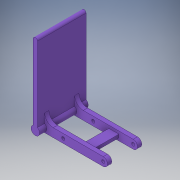
# Autodesk Inventor part: Mouth-Height-Lever-front
Saved by Autodesk Inventor 2018.3 (Build 223284000, 284)
## iProperties
Created: 2018-05-17
Part Number: Mouth-Height-Lever-front
Material: Generisch
Document SubType Name: Modeling
Designer: JochenAlt
Density: 1 g/cm^3
Appearance: Violett
Author: JochenAlt
Autodesk Inventor part; units mm, degrees
ref_plane "YZ Plane" through (0, 0, 0) normal (1, 0, 0) x (0, 1, 0)
ref_plane "XZ Plane" through (0, 0, 0) normal (0, 1, 0) x (-1, 0, 0)
ref_plane "XY Plane" through (0, 0, 0) normal (0, 0, 1) x (1, 0, 0)
sketch "Skizze4" plane through (0, 0, 0) normal (0, 1, 0) x (-1, 0, 0)
  line L0 (-45.5216, 3) -> (-3, 3) construction
  line L1 (0, -14.9) -> (0, 68.4) construction
  line L2 (-58.2259, 0) -> (9.7043, 0) construction
  circle A0 centre (-45.5216, 0) radius 3
  circle A1 centre (-45.5216, 0) radius 1.1
  circle A2 centre (-3, 0) radius 3
  line L3 (-12.1436, -3) -> (-45.5216, -3) construction
  line L4 (-45.5216, -3) -> (-17.5581, -3)
  line L5 (-1.5, 2.5981) -> (-1.5, 55)
  arc A3 (-1.5, 55) -> (-4.5, 55) centre (-3, 55) ccw
  circle A4 centre (-17.5581, 0) radius 1.1
  line L6 (-4.5, 9) -> (-4.5, 55)
  line L7 (-10.5, 3) -> (-3, 3)
  line L8 (-3, 0) -> (-3, 55) construction
  line L9 (-4.5, 9) -> (-4.5, 3)
  arc A5 (-10.5, 3) -> (-4.5, 9) centre (-10.5, 9) ccw
  line L10 (-4.5, 3) -> (-4.5, 2.5981)
  line L11 (-10.5, 3) -> (-10.5, -3)
  line L12 (-10.5, -3) -> (-3, -3)
  line L13 (-10.5, 3) -> (-17.5581, 3)
  line L14 (-10.5, -3) -> (-17.5581, -3)
  arc A6 (-17.5581, -3) -> (-17.5581, 3) centre (-17.5581, 0) ccw
  line L15 (-28.5216, 1.1) -> (-35.5216, 1.1)
  line L16 (-35.5216, 1.1) -> (-35.5216, -1.1)
  line L17 (-35.5216, -1.1) -> (-28.5216, -1.1)
  line L18 (-28.5216, -1.1) -> (-28.5216, 1.1)
  line L19 (-45.5216, 3) -> (-17.5581, 3)
  point P0 (0, 0)
  point P1 (-3, -3)
  point P2 (-3, -3)
  dimension "d35" = 6
  dimension "d28" = 2.2
  dimension "d41" = 3
  dimension "d43" = 55
  dimension "d47" = 10
  dimension "d48" = 6
  constraints: 36 end point, 10 point on circle, 10 tangent, 7 horizontal, 6 centre point, 5 parallel, 4 vertical, 3 perpendicular, 2 coincident, 1 equal radius, 1 point on line, 10 other
  measures "d28" diameter of A1
  measures "d41" distance between parallel lines of L5 L6
  measures "d43" distance from line of L2 L8.end
  measures "d47" distance from line of L16 A0.centre
  measures "d48" radius of A5
extrude "Extrusion6" add sketch "Skizze4" along normal mid plane 24 contours A0 | A0 L19 A6 L4 | L13 L11 L14 A6 | A5 L9 L7 | L7 L10 A2 L12 L11 | L18 L17 L16 L15
extrude "Extrusion8" add sketch "Skizze4" along normal mid plane 34 contours L9 L6 A3 L5 A2 L7 | L7 A2 L10 | A2
extrude "Extrusion7" cut sketch "Skizze4" along normal mid plane 18 contours A0 | A0 L19 A6 L4 | L13 L11 L14 A6 | A5 L9 L7 | L7 L10 A2 L12 L11 | A1
